Autodesk Fusion 360 part; units mm, degrees
(part 2 of 2)
extrude "Extrude14" add 1 faces at (6.154822, -25.624073, 35.232394) along direction (0, 0, -1) blind 12.2174 on bodies 6 bodies 6
extrude "Extrude15" add 1 faces at (1.539589, -24.886565, 24.732394) along direction (0, 0, -1) blind 11 on bodies 6 bodies 6
ref_plane "WorkPlane1" through (0, 0, 0) normal (0, 1, 0) x (0, 0, 1)
ref_plane "WorkPlane2" through (0, 0, 0) normal (0, 1, 0) x (0, 0, 1)
sketch "Sketch10" plane through (0, 0, 0) normal (0, 1, 0) x (1, 0, 0)
  line L0 (6.5125, -59.232503) -> (6.51, -23.015001)
  dimension "d50" = 36.217502
combine "Combine1" [suppressed]
named bodies: "pulley low"

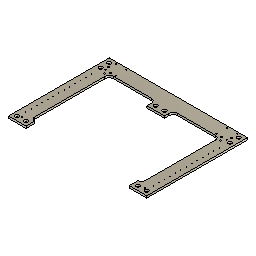
design "top plate for Mark III Corexy"
Autodesk Fusion 360 part; units mm, degrees
sketch "Sketch1" plane through (0, 0, 0) normal (0, 0, 1) x (1, 0, 0)
  line L0 (315.9125, 230.1875) -> (315.9125, -230.1875)
  line L1 (252.4125, 146.6875) -> (252.4125, -175.1875)
  line L2 (-315.9125, -230.1875) -> (-235.9125, -230.1875)
  line L3 (-235.9125, -230.1875) -> (-235.9125, -190.1875)
  line L4 (-235.9125, -190.1875) -> (-237.4125, -190.1875)
  line L5 (235.9125, -230.1875) -> (235.9125, -190.1875)
  line L6 (235.9125, -190.1875) -> (237.4125, -190.1875)
  line L7 (-252.4125, 146.6875) -> (-252.4125, -175.1875)
  arc A0 (-232.4125, 166.6875) -> (-252.4125, 146.6875) centre (-232.4125, 146.6875) ccw
  arc A1 (252.4125, 146.6875) -> (232.4125, 166.6875) centre (232.4125, 146.6875) ccw
  arc A2 (-252.4125, -175.1875) -> (-237.4125, -190.1875) centre (-237.4125, -175.1875) ccw
  arc A3 (237.4125, -190.1875) -> (252.4125, -175.1875) centre (237.4125, -175.1875) ccw
  circle A4 centre (-295.9125, -210.1875) radius 3.5
  circle A5 centre (-255.9125, -210.1875) radius 3.5
  circle A6 centre (255.9125, -210.1875) radius 3.5
  circle A7 centre (295.9125, -210.1875) radius 3.5
  line L8 (40, 126.6875) -> (-40, 126.6875)
  line L9 (40, 126.6875) -> (40, 146.6875)
  line L10 (-40, 126.6875) -> (-40, 146.6875)
  line L11 (-232.4125, 166.6875) -> (-60, 166.6875)
  line L12 (60, 166.6875) -> (232.4125, 166.6875)
  arc A8 (-40, 146.6875) -> (-60, 166.6875) centre (-60, 146.6875) ccw
  arc A9 (60, 166.6875) -> (40, 146.6875) centre (60, 146.6875) ccw
  line L13 (-230.0233, 174.8675) -> (-277.1633, 222.0075) construction
  line L14 (-277.1633, 174.8675) -> (-230.0233, 222.0075) construction
  line L15 (277.1633, 174.8675) -> (230.0233, 222.0075) construction
  line L16 (230.0233, 174.8675) -> (277.1633, 222.0075) construction
  circle A10 centre (-253.5933, 172.8675) radius 8 construction
  circle A11 centre (253.5933, 172.8675) radius 8 construction
  line L17 (315.9125, 192) -> (315.9125, 230.1875) construction
  circle A12 centre (-265, -23) radius 8 construction
  circle A13 centre (265, -22.9937) radius 8 construction
  circle A14 centre (265, 23) radius 8 construction
  circle A15 centre (-281, -203) radius 8 construction
  line L18 (-273, -203) -> (-273, -23) construction
  circle A16 centre (-281, 192) radius 8 construction
  circle A17 centre (-253.5933, 198.4375) radius 8 construction
  line L19 (-281, 200) -> (-255.4853, 206.2105) construction
  line L20 (-247.9364, 192.7806) -> (-259.8461, 177.8577) construction
  circle A18 centre (-264.95, 156.726) radius 8 construction
  circle A19 centre (-264.95, 156.726) radius 3.5
  line L21 (-272.95, 22.9974) -> (-272.95, 156.726) construction
  line L22 (315.9125, 150.1875) -> (315.9125, 230.1875)
  circle A20 centre (253.5933, 198.4375) radius 8 construction
  line L23 (315.9125, 174.8675) -> (315.9125, 230.1875)
  circle A21 centre (253.5933, 172.8675) radius 3.5
  circle A22 centre (-253.5933, 172.8675) radius 3.5
  circle A23 centre (-281, 192) radius 3.5
  circle A24 centre (264.95, 156.6841) radius 3.5
  circle A25 centre (264.95, 156.6841) radius 8 construction
  circle A26 centre (-295.9125, 210.1875) radius 3.5
  circle A27 centre (-295.9125, 170.1875) radius 3.5
  circle A28 centre (295.9125, 210.1875) radius 3.5
  circle A29 centre (295.9125, 170.1875) radius 3.5
  circle A30 centre (-20, 146.6875) radius 3.5
  circle A31 centre (20, 146.6875) radius 3.5
  line L24 (-253.5933, 164.8675) -> (264.9528, 164.6841) construction
  line L25 (272.95, 156.6841) -> (273, 23.003) construction
  line L26 (275, -784) -> (313.5, -784)
  line L27 (-275, -784) -> (-275, -770)
  circle A32 centre (265, -777) radius 8 construction
  line L28 (-255, -770) -> (-255, -790)
  line L29 (236.5, -791.0755) -> (236.5, -790)
  line L30 (-275, -770) -> (-255, -770)
  line L31 (275, -770) -> (255, -770)
  line L32 (252.4125, -790.475) -> (-252.4125, -809.525) construction
  line L33 (255, -790) -> (-255, -790)
  line L34 (261.6667, -790) -> (261.7081, -790.1242) construction
  line L35 (313.5, -816) -> (275, -816)
  line L36 (-275, -784) -> (-313.5, -784)
  line L37 (275, -784) -> (275, -770)
  circle A33 centre (265, -823) radius 8 construction
  line L38 (236.5, -810) -> (236.5, -808.9245)
  line L39 (255, -830) -> (275, -830)
  line L40 (255, -770) -> (255, -790)
  line L41 (-313.5, -784) -> (-313.5, -816)
  circle A34 centre (-265, -823) radius 8 construction
  line L42 (313.5, -784) -> (313.5, -816)
  line L43 (-252.4125, -790.475) -> (252.4125, -809.525) construction
  line L44 (-255, -810) -> (255, -810)
  circle A35 centre (-264.95, -777.0026) radius 8 construction
  line L45 (-313.5, -816) -> (-275, -816)
  line L46 (-255, -830) -> (-275, -830)
  line L47 (255, -810) -> (255, -830)
  line L48 (-255, -810) -> (-255, -830)
  line L49 (-275, -830) -> (-275, -816)
  line L50 (275, -830) -> (275, -816)
  line L51 (235.9125, -230.1875) -> (315.9125, -230.1875)
  line L52 (-315.9125, 230.1875) -> (-315.9125, -230.1875)
  line L53 (315.9125, 230.1875) -> (-315.9125, 230.1875)
  circle A36 centre (281, -203) radius 3.5
  circle A37 centre (281, -203) radius 8 construction
  circle A38 centre (-281, -203) radius 3.5
  circle A39 centre (280.9125, 192) radius 3.5
  circle A40 centre (280.9125, 192) radius 8 construction
  line L54 (289, -203) -> (289, -168) construction
  line L55 (273, -203) -> (273, -22.9937) construction
  circle A41 centre (-264.95, 22.9974) radius 8 construction
  circle A42 centre (-230.0233, 174.8675) radius 2
  circle A43 centre (-230.0233, 222.0075) radius 2
  circle A44 centre (-277.1633, 222.0075) radius 2
  circle A45 centre (-277.1633, 174.8675) radius 2
  circle A46 centre (230.0233, 174.8675) radius 2
  circle A47 centre (277.1633, 174.8675) radius 2
  circle A48 centre (230.0233, 222.0075) radius 2
  circle A49 centre (277.1633, 222.0075) radius 2
  point P0 (-275.9125, -210.1875)
  point P1 (-275.9125, -210.1875)
  point P2 (0, 166.6875)
  point P3 (0, 166.6875)
  point P4 (-253.5933, 198.4375)
  point P5 (253.5933, 198.4375)
  point P6 (-253.5933, 198.4375)
  point P7 (253.5933, 198.4375)
  point P8 (-253.5933, 172.8675)
  point P9 (253.5933, 172.8675)
  point P10 (295.9125, 210.1875)
  point P11 (295.9125, 170.1875)
  point P12 (-295.9125, 170.1875)
  point P13 (-295.9125, 210.1875)
  point P14 (265, 23)
  point P15 (-265, -23)
  point P16 (-265, -23)
  point P17 (265, 23)
  point P18 (265, -22.9937)
  point P19 (265, -22.9937)
  point P20 (-289, 192)
  point P21 (230.0233, 222.0075)
  point P22 (277.1633, 222.0075)
  point P23 (230.0233, 174.8675)
  point P24 (277.1633, 174.8675)
  point P25 (-277.1633, 222.0075)
  point P26 (-230.0233, 222.0075)
  point P27 (-230.0233, 174.8675)
  point P28 (-277.1633, 174.8675)
  point P29 (264.95, 156.6841)
  point P30 (-20, 146.6875)
  point P31 (20, 146.6875)
  point P32 (265, -777)
  point P33 (0, -800)
  point P34 (-275, -800)
  point P35 (265, -823)
  point P36 (-265, -823)
  point P37 (265, -777)
  point P38 (0, -800)
  point P39 (0, -800)
  point P40 (275, -800)
  point P41 (-264.95, -777.0026)
  point P42 (-272.95, -777.0026)
  point P43 (-264.95, -777.0026)
  point P44 (-265, -823)
  point P45 (265, -823)
  point P46 (-273, -823)
  point P47 (-265, -800)
  point P48 (273, -776.997)
  point P49 (281, -203)
  point P50 (280.9125, 192)
  dimension "d1" = 631.825
  dimension "d2" = 460.375
  dimension "d6" = 80
  dimension "d9" = 80
  dimension "d10" = 20
  dimension "d11" = 20
  dimension "d12" = 15
  dimension "d13" = 15
  dimension "d14" = 20
  dimension "d15" = 20
  dimension "d18" = 7
  dimension "d19" = 7
  dimension "d20" = 7
  dimension "d21" = 7
  dimension "d24" = 20
  dimension "d25" = 47.14
  dimension "d26" = 47.14
  dimension "d27" = 47.14
  dimension "d28" = 47.14
  dimension "d30" = 16
  dimension "d31" = 16
  dimension "d32" = 38.1875
  dimension "d35" = 40
  dimension "d39" = 40
  dimension "d50" = 16
  dimension "d51" = 16
  dimension "d52" = 16
  dimension "d54" = 16
  dimension "d57" = 16
  dimension "d58" = 16
  dimension "d59" = 16
  dimension "d60" = 7
  dimension "d65" = 16
  dimension "d69" = 7
  dimension "d70" = 7
  dimension "d71" = 7
  dimension "d76" = 7
  dimension "d77" = 16
  dimension "d78" = 7
  dimension "d79" = 7
  dimension "d80" = 7
  dimension "d81" = 7
  dimension "d85" = 7
  dimension "d86" = 7
  dimension "d87" = 60
  dimension "d88" = 20
  dimension "d89" = 20
  dimension "d90" = 60
  dimension "d91" = 16
  dimension "d92" = 16
  dimension "d93" = 16
  dimension "d94" = 16
  dimension "d98" = 7
  dimension "d99" = 16
  dimension "d100" = 7
  dimension "d105" = 7
  dimension "d106" = 16
  dimension "d344" = 16
  dimension "d565" = 4
  dimension "d566" = 4
  dimension "d567" = 4
  dimension "d568" = 4
  dimension "d569" = 4
  dimension "d570" = 4
  dimension "d571" = 4
  dimension "d572" = 4
  constraint perpendicular L0 L11
  constraint horizontal L2
  constraint vertical L3
  constraint horizontal L4
  constraint vertical L5
  constraint horizontal L6
  constraint tangent L7 A0
  constraint tangent A0 L11
  constraint tangent L1 A1
  constraint tangent A1 L11
  constraint tangent L4 A2
  constraint tangent L7 A2
  constraint tangent L1 A3
  constraint tangent L6 A3
  constraint coincident P1 P0
  constraint horizontal L8
  constraint perpendicular L9 L11
  constraint perpendicular L10 L11
  constraint collinear L11 L12
  constraint coincident P3 L11
  constraint tangent L10 A8
  constraint tangent L11 A8
  constraint tangent L9 A9
  constraint tangent L12 A9
  constraint equal A8 A9
  constraint coincident P3 P2
  constraint coincident L13 P6
  constraint coincident L14 P6
  constraint coincident P6 P4
  constraint coincident L15 P7
  constraint coincident L16 P7
  constraint coincident P7 P5
  constraint coincident P8 A10.centre
  constraint coincident P9 A11.centre
  constraint vertical L17
  constraint coincident P16 P15
  constraint coincident P17 P14
  constraint coincident P19 P18
  constraint coincident A15 L18.start
  constraint coincident A12 L18.end
  constraint tangent A12 L18
  constraint coincident P20 A16
  constraint coincident A16 L19.start
  constraint coincident A17 L19.end
  constraint tangent A17 L19
  constraint coincident A17 L20.start
  constraint coincident L13 L20.start
  constraint coincident A10 L20.end
  constraint tangent A10 L20
  constraint concentric A18 A19
  constraint coincident A18 L21.end
  constraint tangent A18 L21
  constraint vertical L22
  constraint vertical L23
  constraint concentric A11 A21
  constraint concentric A10 A22
  constraint concentric A16 A23
  constraint coincident P21 L15.end
  constraint coincident P22 L16.end
  constraint coincident P23 L16.start
  constraint coincident P24 L15.start
  constraint coincident P25 L13.end
  constraint coincident P26 L14.end
  constraint coincident P27 L13.start
  constraint coincident P28 L14.start
  constraint coincident P29 A24.centre
  constraint coincident P13 A26.centre
  constraint coincident P12 A27.centre
  constraint coincident P10 A28.centre
  constraint coincident P11 A29.centre
  constraint coincident P30 A30.centre
  constraint coincident P31 A31.centre
  constraint coincident A10 L24.start
  constraint coincident A25 L24.end
  constraint tangent A25 L24
  constraint coincident A25 L25.start
  constraint coincident A14 L25.end
  constraint tangent A14 L25
  constraint coincident P39 P38
  constraint coincident P39 L43
  constraint perpendicular L31 L40
  constraint parallel L31 L39
  constraint parallel L40 L50
  constraint horizontal L31
  constraint perpendicular L46 L49
  constraint parallel L30 L46
  constraint parallel L28 L49
  constraint horizontal L46
  constraint horizontal L45
  constraint perpendicular L35 L38
  constraint parallel L38 L42
  constraint horizontal L35
  constraint coincident L38.end L43
  constraint collinear L29 L38
  constraint coincident L38.start L44
  constraint coincident L26.start L50
  constraint coincident L44.end L40
  constraint collinear L37 L50
  constraint coincident P40 L50
  constraint collinear L40 L47
  constraint collinear L27 L49
  constraint coincident P34 L49
  constraint coincident L44.start L28
  constraint collinear L28 L48
  constraint coincident P44 P36
  constraint coincident P43 P41
  constraint coincident P37 P32
  constraint coincident P45 P35
  constraint coincident P46 A34
  constraint coincident P42 A35
  constraint coincident P48 A32
  constraint perpendicular L0 L51
  constraint perpendicular L2 L52
  constraint perpendicular L52 L53
  constraint coincident P49 A36.centre
  constraint concentric A36 A37
  constraint concentric A15 A38
  constraint coincident P50 A39.centre
  constraint coincident A37 L54.start
  constraint tangent A37 L54
  constraint vertical L54
  constraint coincident A37 L55.start
  constraint coincident A13 L55.end
  constraint tangent A13 L55
  constraint vertical L55
  constraint coincident L21.start A41
  measures "d1" distance of L52.start L0.start
  measures "d2" distance of L2.start L52.start
  measures "d6" distance of L2.start L2.end
  measures "d9" distance of L0.end L5.start
  measures "d10" radius of A0
  measures "d11" radius of A1
  measures "d12" radius of A2
  measures "d13" radius of A3
  measures "d14" distance of P1 A5.centre
  measures "d15" distance of P1 A4.centre
  measures "d18" diameter of A4
  measures "d19" diameter of A5
  measures "d20" diameter of A6
  measures "d21" diameter of A7
  measures "d24" radius of A8
  measures "d25" distance of P25 P26
  measures "d26" distance of P28 P25
  measures "d27" distance of P21 P22
  measures "d28" distance of P23 P21
  measures "d30" diameter of A10
  measures "d31" diameter of A11
  measures "d32" distance of L0.start L17.start
  measures "d35" distance of P10 P11
  measures "d39" distance of P12 P13
  measures "d50" diameter of A12
  measures "d51" diameter of A13
  measures "d52" diameter of A14
  measures "d54" diameter of A15
  measures "d57" diameter of A16
  measures "d58" diameter of A17
  measures "d59" diameter of A18
  measures "d60" diameter of A19
  measures "d65" diameter of A20
  measures "d69" diameter of A21
  measures "d70" diameter of A22
  measures "d71" diameter of A23
  measures "d76" diameter of A24
  measures "d77" diameter of A25
  measures "d78" diameter of A26
  measures "d79" diameter of A27
  measures "d80" diameter of A28
  measures "d81" diameter of A29
  measures "d85" diameter of A30
  measures "d86" diameter of A31
  measures "d87" distance of L39.start L31.end
  measures "d88" distance of L39.end L39.start
  measures "d89" distance of L27.end L28.start
  measures "d90" distance of L46.end L27.end
  measures "d91" diameter of A34
  measures "d92" diameter of A33
  measures "d93" diameter of A32
  measures "d94" diameter of A35
  measures "d98" diameter of A36
  measures "d99" diameter of A37
  measures "d100" diameter of A38
  measures "d105" diameter of A39
  measures "d106" diameter of A40
  measures "d344" diameter of A41
  measures "d565" diameter of A42
  measures "d566" diameter of A43
  measures "d567" diameter of A44
  measures "d568" diameter of A45
  measures "d569" diameter of A46
  measures "d570" diameter of A47
  measures "d571" diameter of A48
  measures "d572" diameter of A49
sketch "Sketch2" plane through (0, 0, 0) normal (0, 0, 1) x (1, 0, 0)
extrude "Extrude1" add sketch "Sketch1" along normal blind 9.525 contours L0 L1 L2 L3 L4 L5 L6 L7 A0 A1 A2 A3 L8 L9 L10 L11 L12 A8 A9 L22 L23 L51 L52 L53 | A42 | A43 | A44 | A45 | A46 | A47 | A48 | A49
hole "Hole1" at (277.1633, 222.0075, 0) direction (0, 0, 1) diameter 5 depth 30 tip angle 118
hole "Hole2" at (277.1633, 174.8675, 0) at (230.0233, 174.8675, 0) at (230.0233, 222.0075, 0) direction (0, 0, 1) diameter 5 depth 30 tip angle 118
hole "Hole3" at (-230.0233, 222.0075, 0) at (-230.0233, 174.8675, 0) at (-277.1633, 222.0075, 0) at (-277.1633, 174.8675, 0) direction (0, 0, 1) diameter 5 depth 30 tip angle 118
sketch "Sketch61" plane through (0, 0, 9.525) normal (0, 0, 1) x (-1, 0, 0)
  circle A0 centre (277.1633, -222.0075) radius 2.5
  circle A1 centre (230.0233, -222.0075) radius 2.5
  circle A2 centre (230.0233, -174.8675) radius 2.5
  circle A3 centre (277.1633, -174.8675) radius 2.5
  circle A4 centre (-230.0233, -174.8675) radius 2.5
  circle A5 centre (-277.1633, -174.8675) radius 2.5
  circle A6 centre (-230.0233, -222.0075) radius 2.5
  circle A7 centre (-277.1633, -222.0075) radius 2.5
  circle A8 centre (255.9125, 210.1875) radius 3.5
  circle A9 centre (295.9125, -210.1875) radius 3.5
  circle A10 centre (295.9125, -170.1875) radius 3.5
  circle A11 centre (-295.9125, -210.1875) radius 3.5
  circle A12 centre (295.9125, 210.1875) radius 3.5
  circle A13 centre (-280.9125, -192) radius 3.5
  circle A14 centre (281, 203) radius 3.5
  circle A15 centre (281, -192) radius 3.5
  circle A16 centre (-295.9125, -170.1875) radius 3.5
  circle A17 centre (-295.9125, 210.1875) radius 3.5
  circle A18 centre (-20, -146.6875) radius 3.5
  circle A19 centre (253.5933, -172.8675) radius 3.5
  circle A20 centre (-253.5933, -172.8675) radius 3.5
  circle A21 centre (20, -146.6875) radius 3.5
  circle A22 centre (264.95, -156.726) radius 3.5
  circle A23 centre (-255.9125, 210.1875) radius 3.5
  circle A24 centre (-264.95, -156.6841) radius 3.5
  circle A25 centre (-281, 203) radius 3.5
  line L0 (-315.9125, 230.1875) -> (-315.9125, -230.1875)
  line L1 (-315.9125, -230.1875) -> (315.9125, -230.1875)
  line L2 (315.9125, -230.1875) -> (315.9125, 230.1875)
  line L3 (315.9125, 230.1875) -> (235.9125, 230.1875)
  line L4 (235.9125, 230.1875) -> (235.9125, 190.1875)
  line L5 (235.9125, 190.1875) -> (237.4125, 190.1875)
  arc A26 (252.4125, 175.1875) -> (237.4125, 190.1875) centre (237.4125, 175.1875) ccw
  line L6 (252.4125, 175.1875) -> (252.4125, -146.6875)
  arc A27 (232.4125, -166.6875) -> (252.4125, -146.6875) centre (232.4125, -146.6875) ccw
  line L7 (232.4125, -166.6875) -> (60, -166.6875)
  arc A28 (40, -146.6875) -> (60, -166.6875) centre (60, -146.6875) ccw
  line L8 (40, -146.6875) -> (40, -126.6875)
  line L9 (40, -126.6875) -> (-40, -126.6875)
  line L10 (-40, -126.6875) -> (-40, -146.6875)
  arc A29 (-60, -166.6875) -> (-40, -146.6875) centre (-60, -146.6875) ccw
  line L11 (-60, -166.6875) -> (-232.4125, -166.6875)
  arc A30 (-252.4125, -146.6875) -> (-232.4125, -166.6875) centre (-232.4125, -146.6875) ccw
  line L12 (-252.4125, -146.6875) -> (-252.4125, 175.1875)
  arc A31 (-237.4125, 190.1875) -> (-252.4125, 175.1875) centre (-237.4125, 175.1875) ccw
  line L13 (-237.4125, 190.1875) -> (-235.9125, 190.1875)
  line L14 (-235.9125, 190.1875) -> (-235.9125, 230.1875)
  line L15 (-235.9125, 230.1875) -> (-315.9125, 230.1875)
  point P0 (292, 175)
  point P1 (292, 150)
  point P2 (292, 125)
  point P3 (292, 100)
  point P4 (292, 75)
  point P5 (292, 50)
  point P6 (292, 25)
  point P7 (292, 0)
  point P8 (292, -25)
  point P9 (292, -50)
  point P10 (292, -75)
  point P11 (292, -100)
  point P12 (292, -125)
sketch "Sketch62" plane through (0, 0, 9.525) normal (0, 0, 1) x (-1, 0, 0)
  circle A0 centre (277.1633, -222.0075) radius 2.5
  circle A1 centre (230.0233, -222.0075) radius 2.5
  circle A2 centre (230.0233, -174.8675) radius 2.5
  circle A3 centre (277.1633, -174.8675) radius 2.5
  circle A4 centre (-230.0233, -174.8675) radius 2.5
  circle A5 centre (-277.1633, -174.8675) radius 2.5
  circle A6 centre (-230.0233, -222.0075) radius 2.5
  circle A7 centre (-277.1633, -222.0075) radius 2.5
  circle A8 centre (255.9125, 210.1875) radius 3.5
  circle A9 centre (295.9125, -210.1875) radius 3.5
  circle A10 centre (295.9125, -170.1875) radius 3.5
  circle A11 centre (-295.9125, -210.1875) radius 3.5
  circle A12 centre (295.9125, 210.1875) radius 3.5
  circle A13 centre (-280.9125, -192) radius 3.5
  circle A14 centre (281, 203) radius 3.5
  circle A15 centre (281, -192) radius 3.5
  circle A16 centre (-295.9125, -170.1875) radius 3.5
  circle A17 centre (-295.9125, 210.1875) radius 3.5
  circle A18 centre (-20, -146.6875) radius 3.5
  circle A19 centre (253.5933, -172.8675) radius 3.5
  circle A20 centre (-253.5933, -172.8675) radius 3.5
  circle A21 centre (20, -146.6875) radius 3.5
  circle A22 centre (264.95, -156.726) radius 3.5
  circle A23 centre (-255.9125, 210.1875) radius 3.5
  circle A24 centre (-264.95, -156.6841) radius 3.5
  circle A25 centre (-281, 203) radius 3.5
  line L0 (-315.9125, 230.1875) -> (-315.9125, -230.1875)
  line L1 (-315.9125, -230.1875) -> (315.9125, -230.1875)
  line L2 (315.9125, -230.1875) -> (315.9125, 230.1875)
  line L3 (315.9125, 230.1875) -> (235.9125, 230.1875)
  line L4 (235.9125, 230.1875) -> (235.9125, 190.1875)
  line L5 (235.9125, 190.1875) -> (237.4125, 190.1875)
  arc A26 (252.4125, 175.1875) -> (237.4125, 190.1875) centre (237.4125, 175.1875) ccw
  line L6 (252.4125, 175.1875) -> (252.4125, -146.6875)
  arc A27 (232.4125, -166.6875) -> (252.4125, -146.6875) centre (232.4125, -146.6875) ccw
  line L7 (232.4125, -166.6875) -> (60, -166.6875)
  arc A28 (40, -146.6875) -> (60, -166.6875) centre (60, -146.6875) ccw
  line L8 (40, -146.6875) -> (40, -126.6875)
  line L9 (40, -126.6875) -> (-40, -126.6875)
  line L10 (-40, -126.6875) -> (-40, -146.6875)
  arc A29 (-60, -166.6875) -> (-40, -146.6875) centre (-60, -146.6875) ccw
  line L11 (-60, -166.6875) -> (-232.4125, -166.6875)
  arc A30 (-252.4125, -146.6875) -> (-232.4125, -166.6875) centre (-232.4125, -146.6875) ccw
  line L12 (-252.4125, -146.6875) -> (-252.4125, 175.1875)
  arc A31 (-237.4125, 190.1875) -> (-252.4125, 175.1875) centre (-237.4125, 175.1875) ccw
  line L13 (-237.4125, 190.1875) -> (-235.9125, 190.1875)
  line L14 (-235.9125, 190.1875) -> (-235.9125, 230.1875)
  line L15 (-235.9125, 230.1875) -> (-315.9125, 230.1875)
  point P0 (-292, -125)
  point P1 (-292, -100)
  point P2 (-292, -75)
  point P3 (-292, 0)
  point P4 (-292, -25)
  point P5 (-292, -50)
  point P6 (-292, 25)
  point P7 (-292, 50)
  point P8 (-292, 75)
  point P9 (-292, 100)
  point P10 (-292, 125)
  point P11 (-292, 150)
  point P12 (-292, 175)
hole "Hole50" at (292, 125, 9.525) direction (0, 0, -1) diameter 3 depth 60 tip angle 118
hole "Hole51" at (292, 100, 9.525) at (292, 75, 9.525) at (292, 50, 9.525) at (292, 25, 9.525) at (292, 0, 9.525) at (292, -25, 9.525) at (292, -50, 9.525) at (292, -75, 9.525) at (292, -100, 9.525) at (292, -125, 9.525) at (292, -150, 9.525) at (292, -175, 9.525) at (-292, 125, 9.525) at (-292, 100, 9.525) at (-292, 75, 9.525) at (-292, 50, 9.525) at (-292, 25, 9.525) at (-292, 0, 9.525) at (-292, -25, 9.525) at (-292, -50, 9.525) at (-292, -75, 9.525) at (-292, -100, 9.525) at (-292, -125, 9.525) at (-292, -150, 9.525) at (-292, -175, 9.525) direction (0, 0, -1) diameter 3 depth 60 tip angle 118
chamfer "Chamfer2" distance 5 angle 45 1 edges at (-299.1756, 211.4532, 9.525)
chamfer "Chamfer3" distance 5 angle 45 1 edges at (-299.1756, 171.4532, 9.525)
chamfer "Chamfer4" distance 5 angle 45 8 edges at (-299.1756, -208.9218, 9.525) (-259.1756, -208.9218, 9.525) (292.6494, 211.4532, 9.525) (292.6494, 171.4532, 9.525) (292.6494, -208.9218, 9.525) (252.6494, -208.9218, 9.525) (16.7369, 147.9532, 9.525) (-23.2631, 147.9532, 9.525)
named bodies: "top frame"
